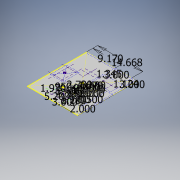
# Autodesk Inventor part: PDU_chassis_bottom
Saved by Autodesk Inventor 2017 (Build 210142000, 142)
## iProperties
Created: 2017-02-14
Part Number: PDU_chassis_bottom
Material: Generic
Document SubType Name: Modeling
Designer: Zara
Density: 1 g/cm^3
Appearance: Default
Author: Zara
Autodesk Inventor part; units mm, degrees
ref_plane "YZ Plane" through (0, 0, 0) normal (1, 0, 0) x (0, 1, 0)
ref_plane "XZ Plane" through (0, 0, 0) normal (0, 1, 0) x (-1, 0, 0)
ref_plane "XY Plane" through (0, 0, 0) normal (0, 0, 1) x (1, 0, 0)
sketch "Sketch1" plane through (0, 0, 0) normal (0, 1, 0) x (-1, 0, 0)
  line L0 (-208.915, 245.999) -> (208.915, 245.999)
  line L1 (208.915, 245.999) -> (208.915, -245.999)
  line L2 (208.915, -245.999) -> (-208.915, -245.999)
  line L3 (-208.915, -245.999) -> (-208.915, 245.999)
  line L4 (-208.915, 245.999) -> (208.915, -245.999) construction
  line L5 (208.915, 245.999) -> (-208.915, -245.999) construction
  point P0 (0, 0)
  dimension "d0" = 491.998
  dimension "d1" = 417.83
  constraints: 12 end point, 2 midpoint, 2 parallel, 1 horizontal, 1 perpendicular
  measures "d0" distance of L2.end L0.start
  measures "d1" distance of L1.end L2.end
extrude "PDU bottom" add sketch "Sketch1" along normal blind 1.651
sketch "Interface circuit board sketch" plane through (0, 1.651, 0) normal (0, 1, 0) x (1, 0, 0)
  line L0 (-208.915, 245.999) -> (-208.915, -245.999) projected
  line L1 (-208.915, -245.999) -> (208.915, -245.999) projected
  point P0 (0, 0)
  point P1 (-50.165, -201.549)
  point P2 (38.735, -201.549)
  point P3 (-50.165, -112.649)
  point P4 (38.735, -112.649)
  dimension "d4" = 158.75
  dimension "d5" = 44.45
  dimension "d9" = 88.9
  dimension "d12" = 88.9
  constraints: 1 horizontal, 1 vertical, 3 other
  measures "d4" distance from line of L0 point (-50.165, -201.549)
  measures "d5" distance from line of point (-50.165, -201.549) L1
  measures "d9" distance of point (-50.165, -201.549) point (38.735, -201.549)
  measures "d12" distance of point (-50.165, -201.549) point (-50.165, -112.649)
sketch "5V monitor psu sketch" plane through (0, 1.651, 0) normal (0, 1, 0) x (1, 0, 0)
  line L0 (-208.915, 245.999) -> (-208.915, -245.999) projected
  line L1 (-208.915, -245.999) -> (208.915, -245.999) projected
  line L2 (17.3991, 155.7782) -> (176.403, 155.7782) construction
  line L3 (176.403, 155.7782) -> (176.403, 58.801) construction
  line L4 (176.403, 58.801) -> (17.3991, 58.801) construction
  line L5 (17.3991, 58.801) -> (17.3991, 155.7782) construction
  line L6 (28.3973, 155.7782) -> (28.3973, 58.801) construction
  point P0 (0, 0)
  point P1 (132.1562, 107.2896)
  point P2 (67.1577, 107.2896)
  dimension "d22" = 341.0712
  dimension "d25" = 276.0727
  dimension "d156" = 48.4886
  dimension "d157" = 48.4886
  dimension "d158" = 49.7586
  dimension "d159" = 44.2468
  dimension "d165" = 10.9982
  dimension "d213" = 353.2886
  dimension "d214" = 353.2886
  constraints: 10 end point, 2 parallel, 2 perpendicular, 2 point on line, 1 horizontal
  measures "d22" distance from line of L0 point (132.156, 107.29)
  measures "d25" distance from line of point (67.158, 107.29) L0
  measures "d156" distance from line of L2 point (67.158, 107.29)
  measures "d157" distance from line of L4 point (67.158, 107.29)
  measures "d158" distance from line of L5 point (67.158, 107.29)
  measures "d159" distance from line of L3 point (132.156, 107.29)
  measures "d165" distance between parallel lines of L6 L5
  measures "d213" distance from line of point (132.156, 107.29) L1
  measures "d214" distance from line of point (67.158, 107.29) L1
sketch "Sketch7" plane through (0, 0, 0) normal (0, -1, 0) x (1, 0, 0)
  line L0 (208.915, 245.999) -> (-208.915, 245.999) projected
  line L1 (-208.915, 245.999) -> (-208.915, -245.999) projected
  line L2 (-208.915, -245.999) -> (208.915, -245.999) projected
  line L3 (208.915, -245.999) -> (208.915, 245.999) projected
  point P0 (0, 0)
  point P1 (-50.165, 112.649)
  point P2 (38.735, 112.649)
  point P3 (38.735, 201.549)
  point P4 (-50.165, 201.549)
hole "Inteface circuit board holes" at (38.735, 0, 112.649) at (-50.165, 0, 112.649) at (-50.165, 0, 201.549) at (38.735, 0, 201.549) direction (0, 1, 0) diameter 3.4036 end through all countersink diameter 6.2992 countersink angle 90
sketch "Sketch9" plane through (0, 0, 0) normal (0, -1, 0) x (1, 0, 0)
  circle A0 centre (-50.165, 201.549) radius 3.1496 projected
  circle A1 centre (38.735, 112.649) radius 3.1496 projected
  circle A2 centre (-50.165, 112.649) radius 3.1496 projected
  circle A3 centre (38.735, 201.549) radius 3.1496 projected
  line L0 (208.915, 245.999) -> (-208.915, 245.999) projected
  line L1 (-208.915, 245.999) -> (-208.915, -245.999) projected
  line L2 (-208.915, -245.999) -> (208.915, -245.999) projected
  line L3 (208.915, -245.999) -> (208.915, 245.999) projected
  point P0 (0, 0)
  point P1 (67.1577, -107.2896)
  point P2 (132.1562, -107.2896)
hole "5V monitor psu holes" at (67.1577, 0, -107.2896) at (132.1562, 0, -107.2896) direction (0, 1, 0) diameter 3.4036 end through all countersink diameter 6.2992 countersink angle 90 clearance for "Countersunk Flat Head Screw ISO 2009/7046" size "M3" standard "ISO"
sketch "thermostat sketch" plane through (0, 1.651, 0) normal (0, 1, 0) x (1, 0, 0)
  line L0 (-47.5742, 118.7155) -> (-47.5742, 94.8903) construction
  line L1 (-208.915, 245.999) -> (-208.915, -245.999) construction
  line L2 (-208.915, -245.999) -> (208.915, -245.999) construction
  point P0 (0, 0)
  dimension "d101" = 161.3408
  dimension "d102" = 364.7145
  dimension "d103" = 23.8252
  constraints: 2 end point, 1 vertical
  measures "d101" distance from line of L1 L0.start
  measures "d102" distance from line of L2 L0.start
  measures "d103" distance of L0.end L0.start
sketch "Sketch11" plane through (0, 0, 0) normal (0, -1, 0) x (1, 0, 0)
  circle A0 centre (67.1577, -107.2896) radius 3.1496 projected
  circle A1 centre (132.1562, -107.2896) radius 3.1496 projected
  circle A2 centre (-50.165, 201.549) radius 3.1496 projected
  circle A3 centre (38.735, 112.649) radius 3.1496 projected
  circle A4 centre (-50.165, 112.649) radius 3.1496 projected
  circle A5 centre (38.735, 201.549) radius 3.1496 projected
  line L0 (208.915, 245.999) -> (-208.915, 245.999) projected
  line L1 (-208.915, 245.999) -> (-208.915, -245.999) projected
  line L2 (-208.915, -245.999) -> (208.915, -245.999) projected
  line L3 (208.915, -245.999) -> (208.915, 245.999) projected
  point P0 (0, 0)
  point P1 (-47.5742, -118.7155)
  point P2 (-47.5742, -94.8903)
hole "thermostat holes" at (-47.5742, 0, -118.7155) at (-47.5742, 0, -94.8903) direction (0, 1, 0) diameter 3.4 end through all countersink diameter 6.3 countersink angle 90 clearance for "Countersunk Flat Head Screw ISO 2009/7046" size "M3" standard "ISO"
sketch "wrlen" plane through (0, 1.651, 0) normal (0, 1, 0) x (1, 0, 0)
  line L0 (-199.39, -236.474) -> (199.39, -236.474) construction
  line L1 (199.39, -236.474) -> (199.39, 236.474) construction
  line L2 (199.39, 236.474) -> (-199.39, 236.474) construction
  line L3 (-199.39, 236.474) -> (-199.39, -236.474) construction
  line L4 (-199.39, -236.474) -> (199.39, 236.474) construction
  line L5 (199.39, -236.474) -> (-199.39, 236.474) construction
  line L6 (208.915, 245.999) -> (-208.915, 245.999) construction
  line L7 (208.915, -245.999) -> (208.915, 245.999) construction
  line L8 (-92.2274, 67.6402) -> (-92.2274, -67.6402) construction
  line L9 (-92.2274, -67.6402) -> (-197.358, -67.6402) construction
  line L10 (-197.358, -67.6402) -> (-197.358, 67.6402) construction
  line L11 (-197.358, 67.6402) -> (-92.2274, 67.6402) construction
  line L12 (-92.2274, 67.6402) -> (-197.358, -67.6402) construction
  line L13 (-92.2274, -67.6402) -> (-197.358, 67.6402) construction
  line L14 (-208.915, -245.999) -> (-208.915, 245.999) construction
  line L15 (-208.915, -245.999) -> (208.915, -245.999) projected
  point P0 (-144.7927, 0)
  point P1 (-144.7927, 0)
  point P2 (-108.1024, 54.9402)
  point P3 (-108.1024, -54.9402)
  point P4 (-174.7774, -54.9402)
  point P5 (-174.7774, 54.9402)
  dimension "d128" = 9.525
  dimension "d129" = 9.525
  dimension "d130" = 105.1306
  dimension "d131" = 135.2804
  dimension "d132" = 15.875
  dimension "d133" = 15.875
  dimension "d134" = 12.7
  dimension "d135" = 12.7
  dimension "d136" = 82.55
  dimension "d137" = 82.55
  dimension "d138" = 12.7
  dimension "d139" = 12.7
  dimension "d140" = 11.557
  dimension "d141" = 178.3588
  constraints: 24 end point, 4 parallel, 3 midpoint, 2 perpendicular, 1 horizontal
  measures "d128" distance between parallel lines of L6 L2
  measures "d129" distance between parallel lines of L1 L7
  measures "d130" distance of L8.end L9.end
  measures "d131" distance of L9.end L13.end
  measures "d132" distance from line of L8 point (-108.102, 54.94)
  measures "d133" distance from line of L8 point (-108.102, -54.94)
  measures "d134" distance from line of point (-108.102, 54.94) L11
  measures "d135" distance from line of L9 point (-108.102, -54.94)
  measures "d136" distance from line of point (-174.777, 54.94) L8
  measures "d137" distance from line of L8 point (-174.777, -54.94)
  measures "d138" distance from line of point (-174.777, 54.94) L11
  measures "d139" distance from line of point (-174.777, -54.94) L9
  measures "d140" distance between parallel lines of L14 L10
  measures "d141" distance between parallel lines of L9 L15
sketch "Sketch15" plane through (0, 0, 0) normal (0, -1, 0) x (1, 0, 0)
  point P0 (0, 0)
  point P1 (-108.1024, -54.9402)
  point P2 (-174.7774, -54.9402)
  point P3 (-174.7774, 54.9402)
  point P4 (-108.1024, 54.9402)
hole "wrlen holes" at (-108.1024, 0, -54.9402) at (-174.7774, 0, -54.9402) at (-174.7774, 0, 54.9402) at (-108.1024, 0, 54.9402) direction (0, 1, 0) diameter 3.4036 end through all countersink diameter 6.2992 countersink angle 90 clearance for "Countersunk Flat Head Screw ISO 2009/7046" size "M3" standard "ISO"
sketch "arduino" plane through (0, 1.651, 0) normal (0, 1, 0) x (1, 0, 0)
  line L0 (8.486, 7.493) -> (111.864, 7.493) construction
  line L1 (111.864, 7.493) -> (111.864, -61.849) construction
  line L2 (111.864, -61.849) -> (8.486, -61.849) construction
  line L3 (8.486, -61.849) -> (8.486, 7.493) construction
  line L4 (33.505, 6.8939) -> (86.845, 6.8939) construction
  line L5 (86.845, 6.8939) -> (86.845, -61.6861) construction
  line L6 (86.845, -61.6861) -> (33.505, -61.6861) construction
  line L7 (33.505, -61.6861) -> (33.505, 6.8939) construction
  point P0 (0, 0)
  point P1 (36.045, -46.609)
  point P2 (51.285, 4.3539)
  point P3 (79.225, 4.3539)
  dimension "d168" = 103.378
  dimension "d169" = 69.342
  dimension "d177" = 68.58
  dimension "d178" = 53.34
  dimension "d179" = 25.019
  dimension "d180" = 15.24
  dimension "d181" = 2.54
  dimension "d182" = 2.54
  dimension "d183" = 2.54
  dimension "d184" = 7.62
  dimension "d185" = 35.56
  constraints: 16 end point, 4 parallel, 2 horizontal, 2 perpendicular
  measures "d168" distance of L0.start L0.end
  measures "d169" distance of L2.end L0.start
  measures "d177" distance of L4.end L5.end
  measures "d178" distance of L5.end L6.end
  measures "d179" distance between parallel lines of L7 L3
  measures "d180" distance from line of point (36.045, -46.609) L2
  measures "d181" distance from line of point (36.045, -46.609) L7
  measures "d182" distance from line of L4 point (51.285, 4.354)
  measures "d183" distance from line of L4 point (79.225, 4.354)
  measures "d184" distance from line of point (79.225, 4.354) L5
  measures "d185" distance from line of point (51.285, 4.354) L5
sketch "power plugs" plane through (0, 1.651, 0) normal (0, 1, 0) x (1, 0, 0)
  line L0 (208.915, 245.999) -> (-208.915, 245.999) construction
  line L1 (58.166, 245.999) -> (24.003, 245.999) construction
  line L2 (24.003, 245.999) -> (24.003, 169.799) construction
  line L3 (24.003, 169.799) -> (58.166, 169.799) construction
  line L4 (58.166, 169.799) -> (58.166, 245.999) construction
  line L5 (-208.915, 245.999) -> (-208.915, -245.999) construction
  line L6 (163.6522, 245.999) -> (192.2018, 245.999) construction
  line L7 (192.2018, 245.999) -> (192.2018, 169.799) construction
  line L8 (192.2018, 169.799) -> (163.6522, 169.799) construction
  line L9 (163.6522, 169.799) -> (163.6522, 245.999) construction
  point P0 (0, 0)
  dimension "d170" = 76.2
  dimension "d172" = 34.163
  dimension "d173" = 232.918
  dimension "d174" = 28.5496
  dimension "d175" = 76.2
  dimension "d176" = 372.5672
  constraints: 16 end point, 4 parallel, 2 horizontal, 2 perpendicular, 2 point on line
  measures "d170" distance of L3.end L1.start
  measures "d172" distance of L2.end L3.end
  measures "d173" distance between parallel lines of L2 L5
  measures "d174" distance of L7.end L8.end
  measures "d175" distance of L6.end L7.end
  measures "d176" distance between parallel lines of L5 L9
sketch "Sketch18" plane through (0, 0, 0) normal (0, -1, 0) x (1, 0, 0)
  point P0 (0, 0)
  point P1 (51.285, -4.3539)
  point P2 (79.225, -4.3539)
  point P3 (36.045, 46.609)
hole "arduino holes" at (51.285, 0, -4.3539) at (36.045, 0, 46.609) at (79.225, 0, -4.3539) direction (0, 1, 0) diameter 2.8956 end through all countersink diameter 5.5118 countersink angle 90 clearance for "Countersunk Flat Head Screw ISO 2009/7046" size "M2.5" standard "ISO"
sketch "snap relay" plane through (0, 1.651, 0) normal (0, 1, 0) x (1, 0, 0)
  line L0 (-74.295, -130.429) -> (62.865, -130.429) construction
  line L1 (62.865, -130.429) -> (62.865, -183.769) construction
  line L2 (62.865, -183.769) -> (-74.295, -183.769) construction
  line L3 (-74.295, -183.769) -> (-74.295, -130.429) construction
  circle A0 centre (38.735, -112.649) radius 1.7018 construction
  line L4 (-74.295, -157.099) -> (62.865, -157.099) construction
  circle A1 centre (-50.165, -112.649) radius 1.7018 construction
  line L5 (-71.755, -182.118) -> (60.325, -182.118) construction
  line L6 (-5.715, -182.118) -> (-5.715, -132.08) construction
  line L7 (-71.9523, -132.08) -> (60.325, -132.08) construction
  point P0 (0, 0)
  point P1 (-71.755, -132.08)
  point P2 (-5.715, -157.099)
  dimension "d193" = 137.16
  dimension "d194" = 53.34
  dimension "d195" = 17.78
  dimension "d196" = 24.13
  dimension "d197" = 132.08
  dimension "d207" = 50.038
  dimension "d208" = 50.038
  dimension "d209" = 132.08
  constraints: 16 end point, 5 midpoint, 3 parallel, 2 coincident, 2 horizontal, 1 perpendicular
  measures "d193" distance of L0.start L0.end
  measures "d194" distance of L0.end L1.end
  measures "d195" distance from line of L0 A0.centre
  measures "d196" distance from line of A1.centre L3
  measures "d197" distance of L5.start L5.end
  measures "d207" distance of L7.end point (60.325, -182.118)
  measures "d208" distance of point (-71.755, -132.08) point (-71.755, -182.118)
  measures "d209" distance of L7.end point (-71.755, -132.08)
sketch "Sketch20" plane through (0, 0, 0) normal (0, -1, 0) x (1, 0, 0)
  point P0 (0, 0)
  point P1 (-71.755, 132.08)
  point P2 (60.325, 132.08)
  point P3 (60.325, 182.118)
  point P4 (-71.755, 182.118)
hole "snap relay holes" at (60.325, 0, 132.08) at (-71.755, 0, 132.08) at (-71.755, 0, 182.118) at (60.325, 0, 182.118) direction (0, 1, 0) diameter 3.4036 end through all countersink diameter 6.2992 countersink angle 90 clearance for "Countersunk Flat Head Screw ISO 2009/7046" size "M3" standard "ISO"
sketch "Sketch21" plane through (0, 1.651, 0) normal (0, 1, 0) x (1, 0, 0)
  line L0 (208.915, 245.999) -> (208.915, -245.999) construction
  line L1 (158.115, 46.101) -> (208.915, 46.101) construction
  line L2 (208.915, 46.101) -> (208.915, -169.799) construction
  line L3 (208.915, -169.799) -> (158.115, -169.799) construction
  line L4 (158.115, -169.799) -> (158.115, 46.101) construction
  line L5 (-208.915, -245.999) -> (208.915, -245.999) construction
  point P0 (0, 0)
  dimension "d210" = 215.9
  dimension "d211" = 50.8
  dimension "d212" = 76.2
  constraints: 8 end point, 2 parallel, 1 horizontal, 1 perpendicular, 1 point on line
  measures "d210" distance of L3.end L1.start
  measures "d211" distance of L2.end L3.end
  measures "d212" distance between parallel lines of L3 L5
body "Solid1"
